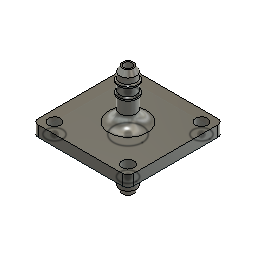
Pneumatic Connectors V1 - O2 V3 (Autodesk Fusion 360 design; units mm, degrees)
Autodesk Fusion 360 part; units mm, degrees
note: some values were not read from the file. Set by a fixed rule: which face or edge a step refers to.
sketch "Sketch1" plane through (0, 0, 0) normal (0, 1, 0) x (1, 0, 0)
  circle A0 centre (0, 0) radius 3
  circle A1 centre (0, 0) radius 1.5
  dimension "d1" = 6
  dimension "d3" = 1.5
  constraint coincident A0.centre A1.centre
  measures "d1" diameter of A0
  measures "d3" distance of A0 A1
extrude "Extrude1" add sketch "Sketch1" along normal blind 18 makes body 1
sketch "Sketch2" plane through (0, 18, 0) normal (0, 1, 0) x (1, 0, 0)
  circle A0 centre (0, 0) radius 1.5
  circle A1 centre (0, 0) radius 3
  line L0 (17.5, 17.5) -> (-17.5, 17.5)
  line L1 (-17.5, 17.5) -> (-17.5, -17.5)
  line L2 (-17.5, -17.5) -> (17.5, -17.5)
  line L3 (17.5, -17.5) -> (17.5, 17.5)
  line L4 (17.5, 17.5) -> (-17.5, -17.5) construction
  line L5 (-17.5, 17.5) -> (17.5, -17.5) construction
  dimension "d6" = 35
  constraint horizontal L0
  constraint perpendicular L0 L1
  constraint parallel L0 L2
  constraint parallel L1 L3
  constraint coincident L4 A0.centre
  constraint coincident L5 A0.centre
  constraint coincident A0.centre A1.centre
  constraint equal L0 L3
  measures "d6" distance of L0.start L0.end
extrude "Extrude2" add sketch "Sketch2" along normal blind 2 contours A1 | L0 L1 L2 L3 bodies 1
ref_plane "WorkPlane1" through (0, 4, 0) normal (0, -1, 0) x (-1, 0, 0)
sketch "Sketch3" plane through (0, 4, 0) normal (0, -1, 0) x (1, 0, 0)
  circle A0 centre (0, 0) radius 3.5
  circle A1 centre (0, 0) radius 3
  dimension "d10" = 0.5
  constraint coincident A0.centre A1.centre
  measures "d10" distance of A0 A1
extrude "Extrude3" add sketch "Sketch3" against normal blind 1 bodies 1
pattern_linear "R-Pattern1" count 2 spacing 4 along (0, 1, 0) of "Extrude3"
chamfer "Chamfer1" distance 0.5 angle 45 2 edges at (-3.2631, 4, -1.2657) (-3.2631, 8, -1.2657) on bodies 1
chamfer "Chamfer2" distance 2 distance2 1 1 edges at (-2.797, 0, 1.0848) measured on face at (2.9851, 2.6667, -0.2987) on bodies 1
mirror "Mirror1" about plane through (0, 20, 0) normal (0, 1, 0) of bodies 1 makes body 2
combine "Combine1" operation add target body 2 tool bodies 1
sketch "Sketch4" plane through (0, 18, 0) normal (0, -1, 0) x (1, 0, 0)
  line L0 (17.5, -17.5) -> (17.5, 17.5) construction
  line L1 (17.5, 17.5) -> (-17.5, 17.5)
  line L2 (-17.5, 17.5) -> (-17.5, -17.5)
  line L3 (-17.5, -17.5) -> (17.5, -17.5)
  line L4 (13.5, 13.5) -> (-13.5, 13.5) construction
  line L5 (-13.5, 13.5) -> (-13.5, -13.5) construction
  line L6 (-13.5, -13.5) -> (13.5, -13.5) construction
  line L7 (13.5, -13.5) -> (13.5, 13.5) construction
  line L8 (13.5, 13.5) -> (-13.5, -13.5) construction
  line L9 (-13.5, 13.5) -> (13.5, -13.5) construction
  circle A0 centre (-13.5, 13.5) radius 2.2
  circle A1 centre (13.5, 13.5) radius 2.2
  circle A2 centre (13.5, -13.5) radius 2.2
  circle A3 centre (-13.5, -13.5) radius 2.2
  circle A4 centre (0, 0) radius 3
  dimension "d22" = 27
  dimension "d23" = 4.4
  constraint horizontal L4
  constraint perpendicular L4 L5
  constraint parallel L4 L6
  constraint parallel L5 L7
  constraint coincident L8 A4.centre
  constraint coincident L9 A4.centre
  constraint equal L4 L7
  constraint coincident L4.end L5.start
  constraint coincident L4.start L7.end
  constraint coincident L6.end L7.start
  constraint coincident L5.end L6.start
  constraint equal A0 A3
  constraint equal A0 A1
  constraint equal A1 A2
  constraint coincident A4.centre origin
  measures "d22" distance of L4.start L4.end
  measures "d23" diameter of A1
fillet "Fillet2" radius 2 4 edges at (17.5, 20, 17.5) (17.5, 20, -17.5) (-17.5, 20, 17.5) (-17.5, 20, -17.5) on bodies 2
extrude "Extrude4" cut sketch "Sketch4" against normal up to surface (4 mm away) contours A0 | A1 | A2 | A3 bodies 2
sketch "Sketch5" plane through (0, 18, 0) normal (0, -1, 0) x (1, 0, 0)
  circle A0 centre (-13.5, 13.5) radius 2.2
  circle A1 centre (13.5, -13.5) radius 2.2
  circle A2 centre (13.5, 13.5) radius 2.2
  circle A3 centre (-13.5, -13.5) radius 2.2
  circle A4 centre (0, 0) radius 3
  arc A5 (-17.5, -15.5) -> (-15.5, -17.5) centre (-15.5, -15.5) ccw
  line L0 (-15.5, -17.5) -> (15.5, -17.5)
  arc A6 (15.5, -17.5) -> (17.5, -15.5) centre (15.5, -15.5) ccw
  line L1 (17.5, -15.5) -> (17.5, 15.5)
  arc A7 (17.5, 15.5) -> (15.5, 17.5) centre (15.5, 15.5) ccw
  line L2 (15.5, 17.5) -> (-15.5, 17.5)
  arc A8 (-15.5, 17.5) -> (-17.5, 15.5) centre (-15.5, 15.5) ccw
  line L3 (-17.5, 15.5) -> (-17.5, -15.5)
  circle A9 centre (0, 0) radius 5
  dimension "d27" = 10
  constraint concentric A4 A9
  measures "d27" diameter of A9
extrude "Extrude5" add sketch "Sketch5" along normal blind 6 contours A9 bodies 2
fillet "Fillet3" radius 4 1 edges at (-2.797, 22, 1.0848) on bodies 2
sketch "Sketch6" plane through (0, 18, 0) normal (0, -1, 0) x (1, 0, 0)
  circle A0 centre (0, 0) radius 5
  circle A1 centre (-13.5, 13.5) radius 2.2
  circle A2 centre (13.5, -13.5) radius 2.2
  circle A3 centre (13.5, 13.5) radius 2.2
  circle A4 centre (-13.5, -13.5) radius 2.2
  arc A5 (-17.5, -15.5) -> (-15.5, -17.5) centre (-15.5, -15.5) ccw
  line L0 (-15.5, -17.5) -> (15.5, -17.5)
  arc A6 (15.5, -17.5) -> (17.5, -15.5) centre (15.5, -15.5) ccw
  line L1 (17.5, -15.5) -> (17.5, 15.5)
  arc A7 (17.5, 15.5) -> (15.5, 17.5) centre (15.5, 15.5) ccw
  line L2 (15.5, 17.5) -> (-15.5, 17.5)
  arc A8 (-15.5, 17.5) -> (-17.5, 15.5) centre (-15.5, 15.5) ccw
  line L3 (-17.5, 15.5) -> (-17.5, -15.5)
  circle A9 centre (0, 0) radius 5.25
  circle A10 centre (-13.5, 13.5) radius 3
  circle A11 centre (13.5, 13.5) radius 3
  circle A12 centre (-13.5, -13.5) radius 3
  circle A13 centre (13.5, -13.5) radius 3
  dimension "d31" = 10.5
  dimension "d32" = 6
  constraint concentric A0 A9
  constraint concentric A1 A10
  constraint concentric A3 A11
  constraint concentric A4 A12
  constraint concentric A2 A13
  constraint equal A11 A13
  constraint equal A10 A11
  constraint equal A10 A12
  measures "d31" diameter of A9
  measures "d32" diameter of A10
equation "d22 = 17 mm + 10 mm"
